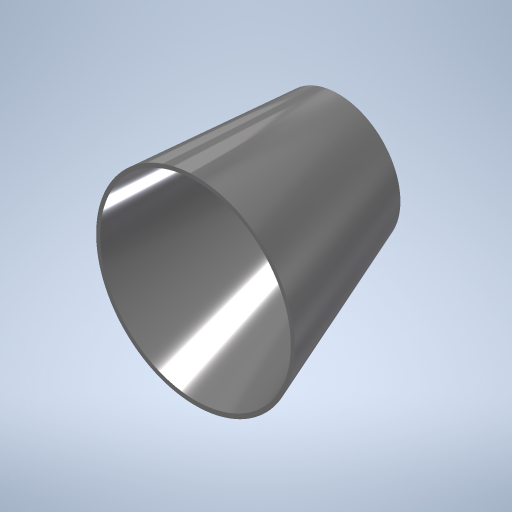
# Autodesk Inventor part: Redukcja asymetryczna Ø101,6x63,5x2 L=73
Saved by Autodesk Inventor 2023 (Build 270158000, 158)
## iProperties
RuleStatus: InUse
Created: 2022-03-21
Part Number: Redukcja asymetryczna Ø101,6x63,5x2 L=73
Material: 304
Description: Redukcja asymetryczna Ø101,6x63,5x2 L=73
Document SubType Name: Modelowanie
Designer: Radosław
Density: 8 g/cm^3
Sheet Metal Rule: 1,5
Sheet Metal Width: 0,000 mm
Sheet Metal Length: 0,000 mm
Sheet Metal Area: 0,000 mm^2
Appearance: Częściowo polerowany(1)
Author: Radosław
Autodesk Inventor part; units mm, degrees
ref_plane "YZ Plane" through (0, 0, 0) normal (1, 0, 0) x (0, 1, 0)
ref_plane "XY Plane" through (0, 0, 0) normal (0, 0, 1) x (1, 0, 0)
sketch "Szkic6" plane through (0, 0, 0) normal (0, 1, 0) x (-1, 0, 0)
  circle A0 centre (0, 0) radius 50.8
  dimension "d33" = 101.6
  constraints: 1 centre point, 1 coincident
  measures "d33" diameter of A0
ref_plane "Płaszczyzna konstrukcyjna1" through (0, 73, 0) normal (0, 1, 0) x (-1, 0, 0)
sketch "Szkic7" plane through (0, 73, 0) normal (0, 1, 0) x (-1, 0, 0)
  circle A0 centre (0, 19.05) radius 31.75
  line L0 (0, -20.3) -> (0, 20.3) construction
  circle A1 centre (0, 0) radius 50.8 construction
  dimension "d35" = 63.5
  constraints: 1 centre point, 1 coincident, 1 point on line, 1 tangent
  measures "d35" diameter of A0
loft "Wyciągnięcie złożone1" add profiles "Szkic6", "Szkic7"
shell "Skorupa1" thickness 2 removed faces 2 at (14.3997, 73, 24.5789) at (7.3018, 0, 11.5135)
equation "\"d33\" = OD1"
equation "\"d35\" = OD2"
equation "\"d52\" = THK"
equation "\"SzerokośćGięciaPodcięcia\" = Grubość"
equation "\"RozmiarPodcięciaNarożnika\" = 4 * Grubość"
equation "\"PromieńPrzejścia\" = PromieńGięcia"
equation "\"Rozmiar_promienia_Jacobiego\" = PromieńGięcia"
equation "\"Wielk_odstępu\" = Grubość"
equation "\"d2\" = PromieńGięcia"
equation "\"d23\" = PromieńGięcia"
equation "\"OD1\" = 101.6"
equation "\"OD2\" = 63.5"
equation "\"L\" = 73"
equation "\"THK\" = 2"
equation "\"d34\" = L"
equation "\"Grubość\" = 1.5"
equation "\"PromieńGięcia\" = 3"
